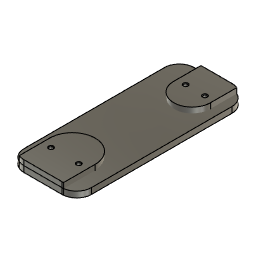
TapAssembly v1 (Autodesk Fusion 360 archive; units mm, degrees)
design "TapMount"
Autodesk Fusion 360 part; units mm, degrees
sketch "Sketch1" plane through (0, 0, 0) normal (0, 0, 1) x (1, 0, 0)
  line L0 (0, 0) -> (0, 440.8206) construction
  circle A0 centre (28.295, 158.91) radius 15.445
  circle A1 centre (34.14, 234.405) radius 12.55
  line L1 (21.59, 252.955) -> (21.59, 225.1955) construction
  line L2 (12.85, 148.5568) -> (12.85, 96.1739) construction
  line L3 (44.5202, 221.855) -> (24.6627, 221.855) construction
  line L4 (16.1034, 174.355) -> (40, 174.355) construction
  line L5 (42.69, 252.955) -> (16.85, 252.955)
  line L6 (6.85, 242.955) -> (6.85, 147.465)
  line L7 (16.85, 137.465) -> (42.69, 137.465)
  line L8 (52.69, 147.465) -> (52.69, 242.955)
  line L9 (46.69, 252.1202) -> (46.69, 234.4206) construction
  line L10 (27.1067, 246.955) -> (40, 246.955) construction
  line L11 (19.6603, 143.465) -> (42.4959, 143.465) construction
  arc A2 (16.85, 252.955) -> (6.85, 242.955) centre (16.85, 242.955) ccw
  arc A3 (42.69, 137.465) -> (52.69, 147.465) centre (42.69, 147.465) ccw
  arc A4 (52.69, 242.955) -> (42.69, 252.955) centre (42.69, 242.955) ccw
  arc A5 (6.85, 147.465) -> (16.85, 137.465) centre (16.85, 147.465) ccw
  line L12 (21.59, 252.955) -> (21.59, 234.405)
  line L13 (46.69, 252.1202) -> (46.69, 234.4206)
  line L14 (12.85, 138.2999) -> (12.85, 158.91)
  line L15 (43.74, 158.91) -> (43.74, 137.465)
  circle A6 centre (18.85, 153.865) radius 1.25
  line L16 (28.295, 158.91) -> (28.295, 137.465)
  circle A7 centre (37.74, 153.865) radius 1.25
  circle A8 centre (40.69, 236.555) radius 1.25
  line L17 (34.14, 234.405) -> (34.14, 252.955)
  circle A9 centre (27.59, 236.555) radius 1.25
  dimension "d1" = 30.89
  dimension "d2" = 25.1
  dimension "d3" = 21.59
  dimension "d4" = 12.85
  dimension "d5" = 47.5
  dimension "d6" = 6
  dimension "d7" = 6
  dimension "d8" = 6
  dimension "d9" = 6
  dimension "d10" = 10
  dimension "d11" = 10
  dimension "d12" = 10
  dimension "d19" = 2.5
  dimension "d20" = 16.4
  dimension "d21" = 12
  dimension "d22" = 2.5
  dimension "d23" = 12
  dimension "d24" = 16.4
  constraint coincident L0.start origin
  constraint vertical L0
  constraint vertical L1
  constraint tangent A1 L1
  constraint vertical L2
  constraint tangent A0 L2
  constraint perpendicular L1 L3
  constraint horizontal L4
  constraint tangent A0 L4
  constraint tangent A1 L3
  constraint horizontal L5
  constraint vertical L6
  constraint horizontal L7
  constraint vertical L8
  constraint vertical L9
  constraint tangent A1 L9
  constraint parallel L5 L10
  constraint tangent A1 L10
  constraint parallel L4 L11
  constraint tangent A0 L11
  constraint tangent L5 A2
  constraint tangent L6 A2
  constraint tangent L7 A3
  constraint tangent L8 A3
  constraint equal A2 A3
  constraint tangent L5 A4
  constraint tangent L8 A4
  constraint tangent L6 A5
  constraint tangent L7 A5
  constraint coincident L5 L1.start
  constraint coincident L1 L12.start
  constraint coincident A1 L12.end
  constraint coincident L1 L12.end
  constraint coincident A4 L9.start
  constraint coincident L9 L13.start
  constraint tangent A1 L13
  constraint coincident A5 L14.start
  constraint coincident L2 L14.start
  constraint coincident A0 L14.end
  constraint tangent A0 L14
  constraint coincident A0 L15.start
  constraint vertical L15
  constraint tangent A0 L15
  constraint coincident A0.centre L16.start
  constraint coincident L7 L16.end
  constraint perpendicular L7 L16
  constraint symmetric A6 L16 A7
  constraint coincident A1.centre L17.start
  constraint coincident L5 L17.end
  constraint perpendicular L5 L17
  constraint symmetric A8 L17 A9
  measures "d1" diameter of A0
  measures "d2" diameter of A1
  measures "d3" distance of L0 L1
  measures "d4" distance of L0 L2
  measures "d5" distance of L3 L4
  measures "d6" distance of L2 L6
  measures "d7" distance of L8 L9
  measures "d8" distance of L5 L10
  measures "d9" distance of L7 L11
  measures "d10" radius of A2
  measures "d11" radius of A4
  measures "d12" radius of A5
  measures "d19" diameter of A6
  measures "d20" distance of L7 A6.centre
  measures "d21" distance of L6 A6.centre
  measures "d22" diameter of A8
  measures "d23" distance of L8 A8.centre
  measures "d24" distance of L5 A8.centre
extrude "Extrude1" add sketch "Sketch1" along normal blind 4 contours A0 | A0 L7 A3 L15 L16 | A0 A1 L5 L6 L8 A2 A3 A4 A5 L12 L13 L14 L15 | A0 L7 A5 L14 L16 | A1 L5 A4 L13 L17 | A1 | A1 L5 L12 L17 | A6 | A7 | A8 | A9 makes body 1
extrude "Extrude2" add sketch "Sketch1" along normal blind 7.5 separate body contours A1 L5 A4 L13 L17 | A1 | A1 L5 L12 L17 | A8 | A9 makes body 2
extrude "Extrude3" add sketch "Sketch1" along normal blind 7.5 separate body contours A0 | A0 L7 A3 L15 L16 | A0 L7 A5 L14 L16 | A6 | A7 makes body 3
extrude "Extrude4" cut sketch "Sketch1" along normal up to surface (7.5 mm away) contours A6 | A7 | A8 | A9 bodies 1 2 3
chamfer "Chamfer1" distance 0.4 angle 45 4 edges at (26.4246, 237.007, 7.5) (39.5246, 237.007, 7.5) (17.6846, 154.317, 7.5) (36.5746, 154.317, 7.5) on bodies 2 3

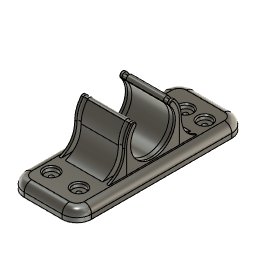
design "TapMountBracket"
Autodesk Fusion 360 part; units mm, degrees
sketch "Sketch1" plane through (0, 0, 0) normal (0, 0, 1) x (1, 0, 0)
  line L0 (0, 0) -> (0, 440.8206) construction
  circle A0 centre (28.295, 158.91) radius 15.445
  circle A1 centre (34.14, 234.405) radius 12.55
  line L1 (21.59, 252.955) -> (21.59, 225.1955) construction
  line L2 (12.85, 148.5568) -> (12.85, 96.1739) construction
  line L3 (44.5202, 221.855) -> (24.6627, 221.855) construction
  line L4 (16.1034, 174.355) -> (40, 174.355) construction
  line L5 (42.69, 252.955) -> (16.85, 252.955)
  line L6 (6.85, 242.955) -> (6.85, 147.465)
  line L7 (16.85, 137.465) -> (42.69, 137.465)
  line L8 (52.69, 147.465) -> (52.69, 242.955)
  line L9 (46.69, 252.1202) -> (46.69, 234.4206) construction
  line L10 (27.1067, 246.955) -> (40, 246.955) construction
  line L11 (19.6603, 143.465) -> (42.4959, 143.465) construction
  arc A2 (16.85, 252.955) -> (6.85, 242.955) centre (16.85, 242.955) ccw
  arc A3 (42.69, 137.465) -> (52.69, 147.465) centre (42.69, 147.465) ccw
  arc A4 (52.69, 242.955) -> (42.69, 252.955) centre (42.69, 242.955) ccw
  arc A5 (6.85, 147.465) -> (16.85, 137.465) centre (16.85, 147.465) ccw
  line L12 (21.59, 252.955) -> (21.59, 234.405)
  line L13 (46.69, 252.1202) -> (46.69, 234.4206)
  line L14 (12.85, 138.2999) -> (12.85, 158.91)
  line L15 (43.74, 158.91) -> (43.74, 137.465)
  circle A6 centre (18.85, 153.865) radius 1.5
  line L16 (28.295, 158.91) -> (28.295, 137.465)
  circle A7 centre (37.74, 153.865) radius 1.5
  circle A8 centre (40.69, 236.555) radius 1.5
  line L17 (34.14, 234.405) -> (34.14, 252.955)
  circle A9 centre (27.59, 236.555) radius 1.5
  circle A10 centre (18.85, 153.865) radius 4.4
  circle A11 centre (37.74, 153.865) radius 4.4
  circle A12 centre (27.59, 236.555) radius 4.4
  circle A13 centre (40.69, 236.555) radius 4.4
  dimension "d1" = 30.89
  dimension "d2" = 25.1
  dimension "d3" = 21.59
  dimension "d4" = 12.85
  dimension "d5" = 47.5
  dimension "d6" = 6
  dimension "d7" = 6
  dimension "d8" = 6
  dimension "d9" = 6
  dimension "d10" = 10
  dimension "d11" = 10
  dimension "d12" = 10
  dimension "d78" = 3
  dimension "d79" = 16.4
  dimension "d80" = 12
  dimension "d81" = 3
  dimension "d82" = 12
  dimension "d83" = 16.4
  dimension "d88" = 8.8
  dimension "d89" = 8.8
  constraint coincident L0.start origin
  constraint vertical L0
  constraint vertical L1
  constraint tangent A1 L1
  constraint vertical L2
  constraint tangent A0 L2
  constraint perpendicular L1 L3
  constraint horizontal L4
  constraint tangent A0 L4
  constraint tangent A1 L3
  constraint horizontal L5
  constraint vertical L6
  constraint horizontal L7
  constraint vertical L8
  constraint vertical L9
  constraint tangent A1 L9
  constraint parallel L5 L10
  constraint tangent A1 L10
  constraint parallel L4 L11
  constraint tangent A0 L11
  constraint tangent L5 A2
  constraint tangent L6 A2
  constraint tangent L7 A3
  constraint tangent L8 A3
  constraint equal A2 A3
  constraint tangent L5 A4
  constraint tangent L8 A4
  constraint tangent L6 A5
  constraint tangent L7 A5
  constraint coincident L5 L1.start
  constraint coincident L1 L12.start
  constraint coincident A1 L12.end
  constraint coincident L1 L12.end
  constraint coincident A4 L9.start
  constraint coincident L9 L13.start
  constraint tangent A1 L13
  constraint coincident A5 L14.start
  constraint coincident L2 L14.start
  constraint coincident A0 L14.end
  constraint tangent A0 L14
  constraint coincident A0 L15.start
  constraint vertical L15
  constraint tangent A0 L15
  constraint coincident A0.centre L16.start
  constraint coincident L7 L16.end
  constraint perpendicular L7 L16
  constraint symmetric A6 L16 A7
  constraint coincident A1.centre L17.start
  constraint coincident L5 L17.end
  constraint perpendicular L5 L17
  constraint symmetric A8 L17 A9
  constraint concentric A6 A10
  constraint symmetric L16 A10 A11
  constraint concentric A9 A12
  constraint symmetric L17 A12 A13
  measures "d1" diameter of A0
  measures "d2" diameter of A1
  measures "d3" distance of L0 L1
  measures "d4" distance of L0 L2
  measures "d5" distance of L3 L4
  measures "d6" distance of L2 L6
  measures "d7" distance of L8 L9
  measures "d8" distance of L5 L10
  measures "d9" distance of L7 L11
  measures "d10" radius of A2
  measures "d11" radius of A4
  measures "d12" radius of A5
  measures "d78" diameter of A6
  measures "d79" distance of L7 A6.centre
  measures "d80" distance of L6 A6.centre
  measures "d81" diameter of A8
  measures "d82" distance of L8 A8.centre
  measures "d83" distance of L5 A8.centre
  measures "d88" diameter of A10
  measures "d89" diameter of A12
extrude "Extrude1" add sketch "Sketch1" along normal blind 4 and the other way blind 4 contours A0 | A0 L7 A3 L15 L16 | A0 A1 L5 L6 L8 A2 A3 A4 A5 L12 L13 L14 L15 | A0 L7 A5 L14 L16 | A1 L5 A4 L13 L17 | A1 | A1 L5 L12 L17 | A6 | A7 | A8 | A9 | A10 | A11 | A12 | A13 makes body 1
ref_plane "WorkPlane1" through (6.85, 195.21, 0) normal (-1, 0, 0) x (0, -1, 0)
sketch "Sketch2" plane through (6.85, 195.21, 2) normal (-1, 0, 0) x (0, 1, 0)
  line L0 (-15.25, -33.5) -> (15.25, -33.5) construction
  line L1 (15.25, -33.5) -> (15.25, -3) construction
  line L2 (15.25, -3) -> (-15.25, -3) construction
  line L3 (-15.25, -3) -> (-15.25, -33.5) construction
  line L4 (-47.745, 2) -> (47.745, 2) construction
  line L5 (0, 2) -> (0, -50) construction
  line L6 (-50, -2) -> (55, -2) construction
  line L7 (-30, -50) -> (-30, -2) construction
  line L8 (30, -50) -> (30, -2) construction
  line L9 (-19.25, -18.25) -> (19.25, -18.25) construction
  spline S0 degree 5 poles (-30, -2) (-29.582, -2.1725) (-28.7638, -2.5309) (-27.59, -3.1088) (-26.1338, -3.961) (-24.5072, -5.1717) (-23.0911, -6.5405) (-21.9021, -8.0798) (-20.9481, -9.7957) (-20.2184, -11.6801) (-19.6956, -13.7198) (-19.4291, -15.4656) (-19.309, -16.8348) (-19.2638, -17.7739) (-19.25, -18.25) knots 0 0 0 0 0 0 0.1 0.2 0.3 0.4 0.5 0.6 0.7 0.8 0.9 1 1 1 1 1 1
  line L10 (15.25, -33.5) -> (-15.25, -33.5) construction
  spline S1 degree 5 poles (30, -2) (29.582, -2.1725) (28.7638, -2.5309) (27.59, -3.1088) (26.1338, -3.961) (24.5072, -5.1717) (23.0911, -6.5405) (21.9021, -8.0798) (20.9481, -9.7957) (20.2184, -11.6801) (19.6956, -13.7198) (19.4291, -15.4656) (19.309, -16.8348) (19.2638, -17.7739) (19.25, -18.25) knots 0 0 0 0 0 0 0.1 0.2 0.3 0.4 0.5 0.6 0.7 0.8 0.9 1 1 1 1 1 1
  line L11 (-32.3433, -1.033) -> (-27.6567, -2.967)
  line L12 (-19.3252, -15.6639) -> (-19.1748, -20.8361)
  line L13 (32.3433, -1.033) -> (27.6567, -2.967)
  line L14 (19.3252, -15.6639) -> (19.1748, -20.8361)
  line L15 (-30, -28) -> (30, -28) construction
  arc A0 (-15.25, -29.9973) -> (-11.726, -28) centre (-13.488, -28.9987) ccw
  arc A1 (11.726, -28) -> (-11.726, -28) centre (0, -18.25) ccw
  arc A2 (11.726, -28) -> (15.25, -29.9973) centre (13.488, -28.9987) ccw
  arc A3 (-19.25, -18.25) -> (-14.8548, -30.4933) centre (0, -18.25) ccw
  arc A4 (14.8548, -30.4933) -> (19.25, -18.25) centre (0, -18.25) ccw
  line L16 (-30, -2) -> (30, -2)
  line L17 (-19.25, -18.25) -> (-19.25, -1.9999) construction
  line L18 (-17.95, -18.25) -> (-17.95, -2)
  arc A5 (-17.95, -18.25) -> (-13.8158, -29.7097) centre (0, -18.25) ccw
  arc A6 (13.8158, -29.7097) -> (17.95, -18.25) centre (0, -18.25) ccw
  line L19 (17.95, -18.25) -> (17.95, -2)
  circle A7 centre (0, -18.25) radius 15.25 construction
  arc A8 (-13.9692, -29.5223) -> (-11.726, -28) centre (-12.8476, -28.7611) ccw
  arc A9 (11.726, -28) -> (13.9692, -29.5223) centre (12.8476, -28.7611) ccw
  point P0 (-22.0357, -8.0113)
  point P1 (22.0357, -8.0113)
  dimension "d20" = 30.5
  dimension "d21" = 5
  dimension "d23" = 4
  dimension "d24" = 30
  dimension "d25" = 30
  dimension "d26" = 25
  dimension "d27" = 1.3
  constraint horizontal L0
  constraint vertical L1
  constraint horizontal L2
  constraint vertical L3
  constraint tangent L0 A1
  constraint tangent L3 A1
  constraint tangent L1 A1
  constraint tangent L2 A1
  constraint midpoint L4 L5.start
  constraint perpendicular L0 L5
  constraint coincident A1.centre L5
  constraint perpendicular L5 L6
  constraint coincident L6 L7.end
  constraint perpendicular L6 L7
  constraint coincident L6 L8.end
  constraint perpendicular L6 L8
  constraint horizontal L9
  constraint midpoint L7.end L11
  constraint midpoint L9.start L12
  constraint symmetric L0.start L5 L0.end
  constraint symmetric L0.end L5 L0.start
  constraint symmetric L5 L7.end L8.end
  constraint symmetric L5 L9.start L9.end
  constraint symmetric L5 P0 P1
  constraint symmetric L5 L11.start L13.start
  constraint symmetric L5 L11.end L13.end
  constraint symmetric L5 L12.start L14.start
  constraint symmetric L5 L12.end L14.end
  constraint coincident L7 L15.start
  constraint coincident L8 L15.end
  constraint perpendicular L8 L15
  constraint coincident L3 A0.start
  constraint coincident L15 A0.end
  constraint coincident A0 A3.end
  constraint coincident L1 A2.end
  constraint coincident L15 A1.start
  constraint coincident A2 A4.start
  constraint concentric A3 A4
  constraint vertical L17
  constraint perpendicular L16 L18
  constraint coincident L6 L18.end
  constraint coincident L9 L18.start
  constraint concentric A4 A5
  constraint tangent L18 A5
  constraint concentric A5 A6
  constraint coincident L9 A6.end
  constraint symmetric L5 L18.start A6.end
  constraint symmetric L5 L18.end L19.end
  constraint concentric A4 A7
  constraint coincident A5 A8.start
  constraint coincident A8 A5.end
  constraint symmetric L5 A0.end A1.start
  constraint symmetric L5 A8.start A9.end
  constraint symmetric L5 A8 A9
  constraint coincident A9 A6.start
  measures "d20" diameter of A1
  measures "d21" distance of L2 L4
  measures "d23" distance of L4 L6
  measures "d24" distance of L5 L7
  measures "d25" distance of L5 L8
  measures "d26" distance of L2 L15
  measures "d27" distance of L17 L18
extrude "Extrude4" add sketch "Sketch2" against normal blind 1.5 from surface at -5.92 separate body contours S0 L12 A0 A3 L16 L18 A5 A8 | L12 A3 | A0 A1 A2 L16 L18 A5 A6 L19 A8 A9 | S1 L14 A2 A4 L16 A6 L19 A9 | L14 A4 makes body 2
extrude "Extrude5" add sketch "Sketch2" against normal blind 34 from surface at -5.92 separate body contours A0 A1 A2 L16 L18 A5 A6 L19 A8 A9 makes body 3
extrude "Extrude6" add sketch "Sketch2" against normal up to surface (25.4 mm away) from surface at -10.22 separate body contours S0 L12 A0 A3 L16 L18 A5 A8 | L12 A3 | A0 A1 A2 L16 L18 A5 A6 L19 A8 A9 | S1 L14 A2 A4 L16 A6 L19 A9 | L14 A4 makes body 4
extrude "Extrude7" add sketch "Sketch2" against normal up to surface (1.5 mm away) from surface at -38.42 separate body contours S0 L12 A0 A3 L16 L18 A5 A8 | L12 A3 | A0 A1 A2 L16 L18 A5 A6 L19 A8 A9 | S1 L14 A2 A4 L16 A6 L19 A9 | L14 A4 makes body 5
ref_plane "WorkPlane2" through (29.77, 195.21, 4) normal (0, 0, 1) x (1, 0, 0)
sketch "Sketch3" plane through (29.77, 195.21, 4) normal (0, 0, 1) x (1, 0, 0)
  line L0 (15.5, -17.95) -> (12.7, -17.95)
  line L1 (22.92, -47.745) -> (22.92, 47.745)
  line L2 (15.5, -17.95) -> (15.5, -19.45)
  line L3 (15.5, -19.45) -> (12.7, -19.45)
  line L4 (12.7, -19.45) -> (12.7, -17.95)
  line L5 (22.92, -17.95) -> (-23, -17.95) construction
  line L6 (0, 0) -> (0, -22.8111)
  line L7 (-15.5, -19.45) -> (-12.7, -19.45)
  line L8 (-12.7, -19.45) -> (-12.7, -17.95)
  line L9 (-15.5, -17.95) -> (-12.7, -17.95)
  line L10 (-15.5, -17.95) -> (-15.5, -19.45)
  line L11 (-19, -0.0001) -> (17, -0.0001)
  line L12 (-15.5, 19.4499) -> (-12.7, 19.4499)
  line L13 (-15.5, 17.9499) -> (-15.5, 19.4499)
  line L14 (-15.5, 17.9499) -> (-12.7, 17.9499)
  line L15 (-12.7, 19.4499) -> (-12.7, 17.9499)
  line L16 (15.5, 19.4499) -> (12.7, 19.4499)
  line L17 (12.7, 19.4499) -> (12.7, 17.9499)
  line L18 (15.5, 17.9499) -> (12.7, 17.9499)
  line L19 (15.5, 17.9499) -> (15.5, 19.4499)
  line L20 (-15.5, 17.9499) -> (-12.7, 17.9499)
  line L21 (-12.7, 17.9499) -> (-12.7, -17.95)
  line L22 (-12.7, -17.95) -> (-15.5, -17.95)
  line L23 (-15.5, -17.95) -> (-15.5, 17.9499)
  line L24 (-15.5, -0.0001) -> (-12.7, -0.0001) construction
  line L25 (12.7, 17.9499) -> (15.5, 17.9499)
  line L26 (15.5, 17.9499) -> (15.5, -17.95)
  line L27 (15.5, -17.95) -> (12.7, -17.95)
  line L28 (12.7, -17.95) -> (12.7, 17.9499)
  line L29 (12.7, -0.0001) -> (15.5, -0.0001) construction
  line L30 (-11.6, -2.5001) -> (-16.6, -2.5001)
  line L31 (-16.6, -2.5001) -> (-16.6, 2.4999)
  line L32 (-16.6, 2.4999) -> (-11.6, 2.4999)
  line L33 (-11.6, 2.4999) -> (-11.6, -2.5001)
  line L34 (-11.6, -2.5001) -> (-16.6, 2.4999) construction
  line L35 (-16.6, -2.5001) -> (-11.6, 2.4999) construction
  line L36 (16.6, -2.5001) -> (11.6, -2.5001)
  line L37 (11.6, -2.5001) -> (11.6, 2.4999)
  line L38 (11.6, 2.4999) -> (16.6, 2.4999)
  line L39 (16.6, 2.4999) -> (16.6, -2.5001)
  line L40 (16.6, -2.5001) -> (11.6, 2.4999) construction
  line L41 (11.6, -2.5001) -> (16.6, 2.4999) construction
  point P0 (-14.1, -0.0001)
  point P1 (14.1, -0.0001)
  point P2 (-14.1, -0.0001)
  point P3 (14.1, -0.0001)
  dimension "d46" = 2.8
  dimension "d47" = 1.5
  dimension "d48" = 7.42
  dimension "d61" = 5
  dimension "d62" = 5
  dimension "d63" = 5
  dimension "d64" = 5
  constraint vertical L2
  constraint vertical L4
  constraint coincident L1 L5.start
  constraint perpendicular L1 L5
  constraint horizontal L0
  constraint collinear L0 L5
  constraint coincident L6.start origin
  constraint symmetric L0.start L6 L9.start
  constraint symmetric L0.end L6 L8.end
  constraint symmetric L2.end L6 L7.start
  constraint symmetric L3.end L6 L7.end
  constraint symmetric L0.start L11 L18.start
  constraint symmetric L0.end L11 L17.end
  constraint symmetric L2.end L11 L16.start
  constraint symmetric L3.end L11 L16.end
  constraint symmetric L7.start L11 L12.start
  constraint symmetric L7.end L11 L12.end
  constraint symmetric L8.end L11 L14.end
  constraint symmetric L9.start L11 L13.start
  constraint horizontal L20
  constraint horizontal L22
  constraint midpoint L23 L24.start
  constraint midpoint L21 L24.end
  constraint midpoint L24 P2
  constraint horizontal L25
  constraint horizontal L27
  constraint vertical L28
  constraint midpoint L28 L29.start
  constraint midpoint L26 L29.end
  constraint midpoint L29 P3
  constraint horizontal L30
  constraint perpendicular L30 L31
  constraint parallel L30 L32
  constraint parallel L31 L33
  constraint coincident L34 P2
  constraint coincident L35 P2
  constraint coincident P2 P0
  constraint horizontal L36
  constraint perpendicular L36 L37
  constraint parallel L36 L38
  constraint parallel L37 L39
  constraint coincident L40 P3
  constraint coincident L41 P3
  constraint coincident P3 P1
  constraint coincident L9.start L10.start
  constraint coincident L14.end L15.end
  measures "d46" distance of L2 L4
  measures "d47" distance of L0 L3
  measures "d48" distance of L1 L2
  measures "d61" distance of L31.end L32.end
  measures "d62" distance of L30.end L31.end
  measures "d63" distance of L37.end L38.end
  measures "d64" distance of L36.end L37.end
extrude "Extrude8" cut sketch "Sketch3" against normal up to surface (8 mm away) contours L7 L8 L9 L10 L22 bodies 1
extrude "Extrude9" cut sketch "Sketch3" against normal up to surface (8 mm away) contours L0 L2 L3 L4 L27 bodies 1
extrude "Extrude10" cut sketch "Sketch3" against normal up to surface (8 mm away) contours L16 L17 L18 L19 L25 | L12 L13 L14 L15 L20 bodies 1
extrude "Extrude11" cut sketch "Sketch3" along normal blind 5.5 from surface at -8 contours L0 L26 L27 L28 L36 | L11 L26 L28 L36 | L11 L26 L36 L39 | L11 L28 L36 L37 | L11 L26 L38 L39 | L11 L26 L28 L38 | L11 L28 L37 L38 | L18 L25 L26 L28 L38 | L9 L21 L22 L23 L30 | L11 L23 L30 L31 | L11 L21 L23 L30 | L11 L21 L30 L33 | L11 L21 L23 L32 | L11 L23 L31 L32 | L11 L21 L32 L33 | L14 L20 L21 L23 L32 bodies 1
fillet "Fillet1" radius 2.5 1 edges at (43.87, 177.26, 1.5) on bodies 1
fillet "Fillet2" radius 2.5 1 edges at (43.87, 213.1599, 1.5) on bodies 1
fillet "Fillet3" radius 2.5 1 edges at (15.67, 177.26, 1.5) on bodies 1
fillet "Fillet4" radius 2.5 1 edges at (15.67, 213.1599, 1.5) on bodies 1
fillet "Fillet5" radius 5 8 edges at (52.69, 195.21, 4) (49.7611, 250.0261, 4) (29.77, 252.955, 4) (9.7789, 250.0261, 4) (6.85, 195.21, 4) (9.7789, 140.3939, 4) (29.77, 137.465, 4) (49.7611, 140.3939, 4) on bodies 1
extrude "Extrude12" cut sketch "Sketch1" along normal up to surface (4 mm away) and the other way up to surface (4 mm away) contours A6 | A7 | A8 | A9 bodies 1
extrude "Extrude13" cut sketch "Sketch1" against normal blind 3 from surface at 4 contours A6 | A7 | A8 | A9 | A10 | A11 | A12 | A13 bodies 1
chamfer "Chamfer1" distance 0.8 angle 45 4 edges at (36.5878, 238.1461, 4) (23.4878, 238.1461, 4) (33.6378, 155.4561, 4) (14.7478, 155.4561, 4) on bodies 1
equation "d32 = -5.92 mm - 1.5 mm - 2.8 mm"
equation "d37 = -1.5 mm - 2.8 mm"
